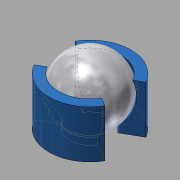
# Autodesk Inventor part: spherical caster ball
Saved by Autodesk Inventor 2015 (Build 190159000, 159)
## iProperties
Created: 2016-10-14
Part Number: spherical caster ball
Material: Generic
Document SubType Name: Modeling
Designer: Paulo Loma
Density: 1 g/cm^3
Appearance: Default
Author: Paulo Loma
Autodesk Inventor part; units mm, degrees
ref_plane "YZ Plane" through (0, 0, 0) normal (1, 0, 0) x (0, 1, 0)
ref_plane "XZ Plane" through (0, 0, 0) normal (0, 1, 0) x (-1, 0, 0)
ref_plane "XY Plane" through (0, 0, 0) normal (0, 0, 1) x (1, 0, 0)
sketch "Sketch1" plane through (0, 0, 0) normal (0, 0, 1) x (1, 0, 0)
  line L0 (-2.5981, -1.5) -> (-1.299, -0.75)
  line L1 (1.299, 0.75) -> (2.5981, 1.5)
  line L2 (-2.5981, 1.5) -> (-1.299, 0.75)
  line L3 (1.299, -0.75) -> (2.5981, -1.5)
  arc A0 (1.299, 0.75) -> (-1.299, 0.75) centre (0, 0) ccw
  arc A1 (-1.299, -0.75) -> (1.299, -0.75) centre (0, 0) ccw
  arc A2 (-2.5981, -1.5) -> (2.5981, -1.5) centre (0, 0) ccw
  arc A3 (2.5981, 1.5) -> (-2.5981, 1.5) centre (0, 0) ccw
  constraints: 8 end point, 8 point on circle, 4 centre point, 3 coincident, 2 other
extrude "Extrusion1" add sketch "Sketch1" along normal blind 1 and the other way blind 2.5
sketch "Sketch4" plane through (0, 0, 0) normal (0, 0, 1) x (1, 0, 0)
  circle A0 centre (0, 0) radius 2.5
  line L0 (2.3998, 0.7008) -> (-2.3998, -0.7008)
  dimension "d8" = 2.5
  constraints: 2 end point, 2 point on circle, 1 centre point, 1 coincident, 1 midpoint
  measures "d8" radius of A0
revolve "Revolution1" add sketch "Sketch4" angle 360 about axis through (2.3998, 0.7008, 0) along (-0.9599048, -0.2803262, 0) separate body picked at (-0.9865, 0.8988) contours L0 A0
combine bodies "Combine1" operation type subtract main body 1 bodies to subtract 2
sketch "Sketch5" plane through (0, 0, 0) normal (0, 0, 1) x (1, 0, 0)
  circle A0 centre (0, 0) radius 2.4
  line L0 (-0.0258, 2.3999) -> (0.0258, -2.3999)
  dimension "d10" = 2.4
  constraints: 2 end point, 2 point on circle, 1 centre point, 1 coincident, 1 midpoint
  measures "d10" radius of A0
revolve "Revolution2" add sketch "Sketch5" angle 360 about axis through (-0.0258, 2.3999, 0) along (0.0107521, -0.9999422, 0) separate body picked at (-1.3089, -0.2294) contours L0 A0
body "Solid3"
body "Solid1"
